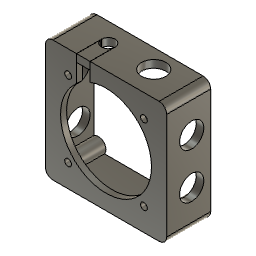
Wanddurchführung (Autodesk Fusion 360 design; units mm, degrees)
Autodesk Fusion 360 part; units mm, degrees
sketch "Sketch1" plane through (0, 0, 0) normal (0, 1, 0) x (1, 0, 0)
  circle A0 centre (0, 0) radius 30
  line L0 (-25, -25) -> (25, -25) construction
  line L1 (25, -25) -> (25, 25) construction
  line L2 (25, 25) -> (-25, 25) construction
  line L3 (-25, 25) -> (-25, -25) construction
  line L4 (0, 0) -> (0, -25) construction
  line L5 (0, 0) -> (25, 0) construction
  circle A1 centre (-25, -25) radius 2.25
  circle A2 centre (25, -25) radius 2.25
  circle A3 centre (25, 25) radius 2.25
  circle A4 centre (-25, 25) radius 2.25
  line L6 (-40, -40) -> (40, -40)
  line L7 (40, -40) -> (40, 40)
  line L8 (40, 40) -> (-40, 40)
  line L9 (-40, 40) -> (-40, -40)
  line L10 (-35, -35) -> (35, -35)
  line L11 (35, -35) -> (35, 35)
  line L12 (35, 35) -> (-35, 35)
  line L13 (-35, 35) -> (-35, -35)
  line L14 (-37, -37) -> (37, -37)
  line L15 (37, -37) -> (37, 37)
  line L16 (37, 37) -> (-37, 37)
  line L17 (-37, 37) -> (-37, -37)
  line L18 (-37.5, -37.5) -> (37.5, -37.5)
  line L19 (37.5, -37.5) -> (37.5, 37.5)
  line L20 (37.5, 37.5) -> (-37.5, 37.5)
  line L21 (-37.5, 37.5) -> (-37.5, -37.5)
  circle A5 centre (-25, -25) radius 5 construction
  circle A6 centre (32.0711, -32.0711) radius 5
  line L22 (32.0711, -32.0711) -> (-32.0711, -32.0711) construction
  line L23 (-32.0711, -32.0711) -> (-32.0711, 32.0711) construction
  line L24 (-32.0711, 32.0711) -> (32.0711, 32.0711) construction
  line L25 (32.0711, 32.0711) -> (32.0711, -32.0711) construction
  circle A7 centre (-32.0711, -32.0711) radius 5
  circle A8 centre (-32.0711, 32.0711) radius 5
  circle A9 centre (32.0711, 32.0711) radius 5
  circle A10 centre (25, -25) radius 5 construction
  circle A11 centre (32.0711, -32.0711) radius 2.75
  circle A12 centre (-32.0711, -32.0711) radius 2.75
  circle A13 centre (32.0711, 32.0711) radius 2.75
  circle A14 centre (-32.0711, 32.0711) radius 2.75
  circle A15 centre (32.0711, 32.0711) radius 2.25
  circle A16 centre (-32.0711, 32.0711) radius 2.25
  circle A17 centre (-32.0711, -32.0711) radius 2.25
  circle A18 centre (32.0711, -32.0711) radius 2.25
  dimension "d1" = 60
  dimension "d2" = 4.5
  dimension "d5" = 50
  dimension "d6" = 80
  dimension "d7" = 5
  dimension "d8" = 2
  dimension "d9" = 0.5
  dimension "d10" = 10
  dimension "d34" = 10
  dimension "d35" = 10
  dimension "d36" = 5.5
  dimension "d37" = 4.5
  constraint coincident A0.centre L4.start
  constraint horizontal L0
  constraint vertical L1
  constraint horizontal L2
  constraint vertical L3
  constraint midpoint L0 L4.end
  constraint midpoint L1 L5.end
  constraint vertical L4
  constraint horizontal L5
  constraint equal L0 L1
  constraint coincident L0.start L3.end
  constraint coincident L0.end L1.start
  constraint coincident L1.end L2.start
  constraint coincident L2.end L3.start
  constraint equal A1 A2
  constraint equal A2 A3
  constraint equal A3 A4
  constraint horizontal L6
  constraint vertical L7
  constraint horizontal L8
  constraint vertical L9
  constraint symmetric L4 L6.start L6.end
  constraint symmetric L5 L6.end L7.end
  constraint equal L6 L7
  constraint horizontal L10
  constraint vertical L11
  constraint horizontal L12
  constraint vertical L13
  constraint symmetric L4 L10.start L10.end
  constraint symmetric L5 L10.end L11.end
  constraint equal L10 L11
  constraint horizontal L14
  constraint vertical L15
  constraint horizontal L16
  constraint vertical L17
  constraint symmetric L4 L14.start L14.end
  constraint symmetric L5 L14.end L15.end
  constraint equal L14 L15
  constraint horizontal L18
  constraint vertical L19
  constraint horizontal L20
  constraint vertical L21
  constraint symmetric L4 L18.start L18.end
  constraint symmetric L5 L18.end L19.end
  constraint equal L18 L19
  constraint concentric A1 A5
  constraint horizontal L22
  constraint vertical L23
  constraint horizontal L24
  constraint vertical L25
  constraint coincident A6.centre L22.start
  constraint symmetric L4 A6.centre L22.end
  constraint symmetric L5 L22.end L23.end
  constraint equal L22 L23
  constraint coincident L22.end L23.start
  constraint coincident L23.end L24.start
  constraint coincident L24.end L25.start
  constraint equal A6 A9
  constraint equal A8 A9
  constraint equal A7 A8
  constraint concentric A2 A10
  constraint tangent A6 A10
  constraint concentric A6 A11
  constraint concentric A7 A12
  constraint concentric A9 A13
  constraint concentric A8 A14
  constraint equal A11 A12
  constraint equal A12 A14
  constraint equal A13 A14
  constraint concentric A13 A15
  constraint concentric A8 A16
  constraint concentric A12 A17
  constraint concentric A11 A18
  constraint equal A15 A18
  constraint equal A15 A16
  constraint equal A16 A17
  measures "d1" diameter of A0
  measures "d2" diameter of A1
  measures "d5" distance of L0.start L0.end
  measures "d6" distance of L6.start L6.end
  measures "d7" vertical distance of L6.start L10.start
  measures "d8" vertical distance of L10.start L14.start
  measures "d9" distance of L14 L18
  measures "d10" diameter of A5
  measures "d34" diameter of A6
  measures "d35" diameter of A10
  measures "d36" diameter of A11
  measures "d37" diameter of A16
extrude "Extrude1" add sketch "Sketch1" along normal blind 4 contours L6 L7 L8 L9 | L10 L13 A7 | L10 L13 L14 L17 A7 | L10 L11 L12 L13 A6 A7 A8 A9 | L10 L14 A6 A7 | L13 L17 A7 A8 | L10 L11 A6 | L10 L11 L14 L15 A6 | L14 A7 | L12 L13 L16 L17 A8 | L12 L13 A8 | L17 A7 | L11 L15 A6 A9 | L14 A6 | L14 L17 A7 | L17 A8 | L11 L12 A9 | L11 L12 L15 L16 A9 | L15 A6 | L14 L15 A6 | L12 L16 A8 A9 | L16 L17 A8 | L15 A9 | L16 A8 | L16 A9 | L15 L16 A9 | L18 L19 L20 L21 | A11 | A12 | A13 | A14 | A15 | A16 | A17 | A18 makes body 1
extrude "Extrude2" add sketch "Sketch1" along normal blind 29 contours L6 L7 L8 L9 | L10 L13 A7 | L10 L13 L14 L17 A7 | L10 L14 A6 A7 | L13 L17 A7 A8 | L10 L11 A6 | L10 L11 L14 L15 A6 | L14 A7 | L12 L13 L16 L17 A8 | L12 L13 A8 | L17 A7 | L11 L15 A6 A9 | L14 A6 | L14 L17 A7 | L17 A8 | L11 L12 A9 | L11 L12 L15 L16 A9 | L15 A6 | L14 L15 A6 | L12 L16 A8 A9 | L16 L17 A8 | L15 A9 | L16 A8 | L16 A9 | L15 L16 A9 | L18 L19 L20 L21 bodies 1
sketch "Sketch2" plane through (-40, 0, 0) normal (-1, 0, 0) x (0, -1, 0)
  line L0 (0, -40) -> (0, 40)
  line L1 (0, 40) -> (-29, 40)
  line L2 (-29, 40) -> (-29, -40)
  line L3 (-29, -40) -> (0, -40)
  line L4 (0, 0) -> (-29, 0) construction
  line L5 (-16.5, -40) -> (-16.5, 40) construction
  circle A0 centre (-16.5, -15) radius 8
  circle A1 centre (-16.5, -15) radius 11 construction
  circle A2 centre (-16.5, 15) radius 11 construction
  circle A3 centre (-16.5, 15) radius 8
  point P0 (-14.5, 40)
  dimension "d15" = 16
  dimension "d16" = 22
  dimension "d17" = 30
  dimension "d54" = 2
  constraint coincident L4.start origin
  constraint midpoint L2 L4.end
  constraint coincident L5 A0.centre
  constraint concentric A0 A1
  constraint coincident L5 A2.centre
  constraint concentric A2 A3
  constraint equal A0 A3
  constraint equal A1 A2
  constraint symmetric L4 A0.centre A2.centre
  constraint coincident L1 L5.end
  constraint midpoint L1 P0
  measures "d15" diameter of A0
  measures "d16" diameter of A1
  measures "d17" distance of A0.centre A2.centre
  measures "d54" distance of L5.end P0
extrude "Extrude3" cut sketch "Sketch2" against normal blind 95 contours A0 | A3 bodies 1
sketch "Sketch3" plane through (0, 0, 40) normal (0, 0, 1) x (-1, 0, 0)
  line L0 (40, 0) -> (-40, 0)
  line L1 (-40, 0) -> (-40, -29)
  line L2 (-40, -29) -> (40, -29)
  line L3 (40, -29) -> (40, 0)
  line L4 (40, -16.5) -> (-40, -16.5) construction
  line L5 (0, -29) -> (0, 0) construction
  circle A0 centre (15, -16.5) radius 4.5
  circle A1 centre (-15, -16.5) radius 8
  line L6 (19.5, -16.5) -> (19.5, 0)
  line L7 (10.5, -16.5) -> (10.5, 0)
  line L8 (40, -27.5) -> (40, -5.5)
  point P0 (40, -14.5)
  dimension "d21" = 30
  dimension "d40" = 16
  dimension "d41" = 9
  dimension "d55" = 2
  constraint midpoint L2 L5.start
  constraint coincident L5.end origin
  constraint coincident L4 A0.centre
  constraint coincident L4 A1.centre
  constraint symmetric L5 A0.centre A1.centre
  constraint coincident A0 L6.start
  constraint coincident L4 L6.start
  constraint coincident L0 L6.end
  constraint tangent A0 L6
  constraint coincident A0 L7.start
  constraint coincident L4 L7.start
  constraint coincident L0 L7.end
  constraint tangent A0 L7
  constraint coincident L1 L4.end
  constraint midpoint L3 P0
  constraint coincident L4.start L8
  measures "d21" distance of A0.centre A1.centre
  measures "d40" diameter of A1
  measures "d41" diameter of A0
  measures "d55" distance of L4.start P0
extrude "Extrude4" cut sketch "Sketch3" against normal blind 28 contours L0 A0 L6 L7 | A0 | A1 bodies 1
extrude "Extrude5" cut sketch "Sketch1" against normal blind 2 from surface at 29 contours L10 L13 A7 | L10 L13 L14 L17 A7 | L10 L14 A6 A7 | L13 L17 A7 A8 | L10 L11 A6 | L10 L11 L14 L15 A6 | L14 A7 | L12 L13 L16 L17 A8 | L12 L13 A8 | L17 A7 | L11 L15 A6 A9 | L14 A6 | L14 L17 A7 | L17 A8 | L11 L12 A9 | L11 L12 L15 L16 A9 | L15 A6 | L14 L15 A6 | L12 L16 A8 A9 | L16 L17 A8 | L15 A9 | L16 A8 | L16 A9 | L15 L16 A9 | L18 L19 L20 L21 bodies 1
extrude "Extrude6" add sketch "Sketch1" along normal blind 4 from surface at 29 separate body contours A0 | A1 | A2 | A3 | A4 | L6 L7 L8 L9 | L10 L13 A7 | L10 L13 L14 L17 A7 | L10 L11 L12 L13 A6 A7 A8 A9 | L10 L14 A6 A7 | L13 L17 A7 A8 | L10 L11 A6 | L10 L11 L14 L15 A6 | L14 A7 | L12 L13 L16 L17 A8 | L12 L13 A8 | L17 A7 | L11 L15 A6 A9 | L14 A6 | L14 L17 A7 | L17 A8 | L11 L12 A9 | L11 L12 L15 L16 A9 | L15 A6 | L14 L15 A6 | L12 L16 A8 A9 | L16 L17 A8 | L15 A9 | L16 A8 | L16 A9 | L15 L16 A9 | L18 L19 L20 L21 | A11 | A12 | A13 | A14 makes body 2
extrude "Extrude7" add sketch "Sketch1" against normal blind 1.8 from surface at 29 contours L10 L13 L14 L17 A7 | L10 L14 A6 A7 | L13 L17 A7 A8 | L10 L11 L14 L15 A6 | L12 L13 L16 L17 A8 | L11 L15 A6 A9 | L14 L17 A7 | L11 L12 L15 L16 A9 | L14 L15 A6 | L12 L16 A8 A9 | L16 L17 A8 | L15 L16 A9 bodies 2
chamfer "Chamfer1" distance 1 angle 45 4 edges at (-27.0977, 4, 24.1864) (-27.0977, 4, -25.8136) (22.9023, 4, 24.1864) (22.9023, 4, -25.8136) on bodies 1
fillet "Fillet1" radius 5 8 edges at (-40, 14.5, -40) (-40, 14.5, 40) (40, 14.5, -40) (40, 14.5, 40) (-40, 31, -40) (-40, 31, 40) (40, 31, -40) (40, 31, 40) on bodies 1 2
extrude "Extrude8" add sketch "Sketch3" against normal blind 5 separate body contours L0 A0 L6 L7 makes body 3
extrude "Extrude9" cut 1 faces at (-10.5, 11, 38.3333) along direction (-1, 0, 0) blind 0.1 on bodies 3 bodies 3
extrude "Extrude10" cut 1 faces at (-19.5, 11, 38.3333) along direction (1, 0, 0) blind 0.1 on bodies 3 bodies 3
sketch "Sketch4" plane through (0, 0, 35) normal (0, 0, -1) x (1, 0, 0)
  line L0 (-19.4, 0) -> (-19.4, -15.5566)
  arc A0 (-10.6, -15.5566) -> (-19.4, -15.5566) centre (-15, -16.5) ccw
  line L1 (-10.6, -15.5566) -> (-10.6, 0)
  line L2 (-10.6, 0) -> (-19.4, 0)
  line L3 (-20.4, -4.1) -> (-9.6, -4.1)
  line L4 (-9.6, -4.1) -> (-9.6, -8.1)
  line L5 (-9.6, -8.1) -> (-20.4, -8.1)
  line L6 (-20.4, -8.1) -> (-20.4, -4.1)
  point P0 (-19.4, -8.1)
  point P1 (-10.6, -8.1)
  dimension "d48" = 4.1
  dimension "d49" = 1
  dimension "d50" = 1
  dimension "d51" = 4
  constraint horizontal L3
  constraint vertical L4
  constraint horizontal L5
  constraint vertical L6
  constraint coincident L0 P0
  constraint coincident L5 P0
  constraint coincident L5 P1
  constraint coincident L1 P1
  measures "d48" distance of L0.start L3
  measures "d49" distance of L5.end P0
  measures "d50" distance of L4.end P1
  measures "d51" distance of L3.end L4.end
extrude "Extrude11" add sketch "Sketch4" along normal blind 1 contours L0 L1 L3 L5 | L0 L3 L5 L6 | L1 L3 L4 L5 bodies 3
hidden bodies 2
equation "d21 = d17"
equation "d40 = d15"
named bodies: "Wanddurchführung_bot", "Wanddurchführung_top", "Wanddurchführung_cap"
